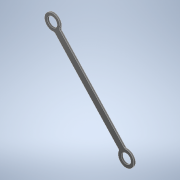
# Autodesk Inventor part: Pieza8
Saved by Autodesk Inventor 2022 (Build 260153000, 153)
## iProperties
Created: 2022-11-04
Part Number: Pieza8
Material: Resina acetálica, negra
Document SubType Name: Modeling
Designer: Mauricio Guerrero
Density: 1.425 g/cm^3
Appearance: Suave - Negro
Author: Mauricio Guerrero
Autodesk Inventor part; units mm, degrees
ref_plane "YZ Plane" through (0, 0, 0) normal (1, 0, 0) x (0, 1, 0)
ref_plane "XZ Plane" through (0, 0, 0) normal (0, 1, 0) x (-1, 0, 0)
ref_plane "XY Plane" through (0, 0, 0) normal (0, 0, 1) x (1, 0, 0)
sketch "Boceto1" plane through (0, 0, 0) normal (0, 0, 1) x (1, 0, 0)
  circle A0 centre (684.3626, 308.7393) radius 1.25
  arc A1 (686.3, 308.204) -> (684.6457, 306.7493) centre (684.3626, 308.7393) ccw
  circle A2 centre (703.3626, 287.7393) radius 1.25
  arc A3 (701.465, 288.4881) -> (703.281, 289.7777) centre (703.3626, 287.7393) ccw
  line L0 (684.3626, 308.7393) -> (703.3626, 287.7393) construction
  line L1 (689.4053, 303.1658) -> (691.9544, 305.4721) construction
  line L2 (686.4151, 307.7311) -> (702.8942, 289.9375)
  line L3 (685.0829, 306.5941) -> (701.3667, 289.0114)
  arc A4 (702.8942, 289.9375) -> (703.281, 289.7777) centre (703.261, 290.2773) ccw
  arc A5 (701.465, 288.4881) -> (701.3667, 289.0114) centre (700.9999, 288.6716) ccw
  arc A6 (686.3, 308.204) -> (686.4151, 307.7311) centre (686.782, 308.0708) ccw
  arc A7 (685.0829, 306.5941) -> (684.6457, 306.7493) centre (684.7161, 306.2543) ccw
  point P0 (0, 0)
  point P1 (685.216, 309.1769)
  point P2 (703.1674, 288.8662)
  point P3 (683.8421, 307.9339)
  point P4 (702.2609, 288.0459)
  point P5 (686.2115, 307.9509)
  point P6 (684.8919, 306.8003)
  point P7 (701.5976, 288.7621)
  point P8 (703.0614, 289.757)
  dimension "d7" = 2.5
  dimension "d8" = 4.02
  dimension "d10" = 4.08
  dimension "d11" = 19
  dimension "d12" = 21
  dimension "d14" = 1.75
  dimension "d15" = 0.5
  constraints: 16 point on circle, 8 centre point, 8 end point, 8 tangent, 5 point on line, 3 equal radius, 2 coincident, 2 symmetric about line, 1 perpendicular
  measures "d7" diameter of A0
  measures "d8" diameter of A1
  measures "d10" diameter of A3
  measures "d11" horizontal distance of A2.centre A0.centre
  measures "d12" vertical distance of A2.centre A0.centre
  measures "d14" distance between parallel lines of L2 L3
  measures "d15" radius of A4
extrude "Extrusión1" add sketch "Boceto1" along normal blind 0.4
